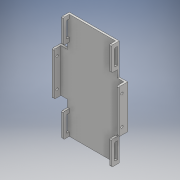
# Autodesk Inventor part: RCT-H112_stick_battery_plate
Saved by Autodesk Inventor 2018.1 (Build 221171000, 171)
## iProperties
Created: 2019-09-19
Part Number: RCT-H112_stick_battery_plate
Material: Generic
Document SubType Name: Modeling
Designer: maste
Density: 1 g/cm^3
Appearance: Default
Author: maste
Autodesk Inventor part; units mm, degrees
ref_plane "YZ Plane" through (0, 0, 0) normal (1, 0, 0) x (0, 1, 0)
ref_plane "XZ Plane" through (0, 0, 0) normal (0, 1, 0) x (-1, 0, 0)
ref_plane "XY Plane" through (0, 0, 0) normal (0, 0, 1) x (1, 0, 0)
sketch "Sketch1" plane through (0, 0, 0) normal (0, 1, 0) x (-1, 0, 0)
  line L0 (34.75, 22.5) -> (34.75, -22.5)
  line L1 (-34.75, 22.5) -> (-34.75, -22.5)
  line L2 (34.75, -22.5) -> (26, -22.5)
  line L3 (-34.75, -22.5) -> (-26, -22.5)
  line L4 (34.75, 22.5) -> (26, 22.5)
  line L5 (-34.75, 22.5) -> (-26, 22.5)
  line L6 (-26, -22.5) -> (-26, -55)
  line L7 (26, -22.5) -> (26, -55)
  line L8 (26, 22.5) -> (26, 55)
  line L9 (-26, 22.5) -> (-26, 55)
  line L10 (26, 55) -> (-26, 55)
  line L11 (26, -55) -> (-26, -55)
  point P0 (0, 0)
  dimension "d0" = 45
  dimension "d1" = 34.75
  dimension "d2" = 22.5
  dimension "d3" = 45
  dimension "d4" = 34.75
  dimension "d5" = 22.5
  dimension "d6" = 8.75
  dimension "d7" = 8.75
  dimension "d8" = 8.75
  dimension "d9" = 8.75
  dimension "d10" = 32.5
  dimension "d11" = 32.5
  dimension "d12" = 32.5
  dimension "d13" = 32.5
  constraints: 24 end point, 6 vertical, 4 horizontal
  measures "d0" distance of L0.start L0.end
  measures "d1" distance from line of point (0, 0) L0
  measures "d2" vertical distance of point (0, 0) L0.start
  measures "d3" distance of L1.start L1.end
  measures "d4" distance from line of point (0, 0) L1
  measures "d5" vertical distance of point (0, 0) L1.start
  measures "d6" distance of L0.end L2.end
  measures "d7" distance of L1.end L3.end
  measures "d8" distance of L0.start L4.end
  measures "d9" distance of L1.start L5.end
  measures "d10" distance of L3.end L6.end
  measures "d11" distance of L2.end L7.end
  measures "d12" distance of L4.end L8.end
  measures "d13" distance of L5.end L9.end
extrude "Extrusion1" add sketch "Sketch1" along normal blind 2
sketch "Sketch2" plane through (34.75, 0, 22.5) normal (1, 0, 0) x (0, 0, -1)
  line L0 (45, 2) -> (77.5, 2) projected
  line L1 (45, 2) -> (0, 2) projected
  line L2 (45, 2) -> (0, 2)
  line L3 (0, 2) -> (0, -6)
  line L4 (1, -7) -> (44, -7)
  line L5 (45, -6) -> (45, 2)
  line L6 (7.5, -4) -> (37.5, -4) construction
  circle A0 centre (7.5, -4) radius 1.25
  circle A1 centre (37.5, -4) radius 1.25
  arc A2 (0, -6) -> (1, -7) centre (1, -6) ccw
  arc A3 (44, -7) -> (45, -6) centre (44, -6) ccw
  point P0 (22.5, 0)
  point P1 (0, -7)
  point P2 (45, -7)
  dimension "d16" = 9
  dimension "d17" = 45
  dimension "d18" = 30
  dimension "d19" = 3
  dimension "d20" = 7.5
  dimension "d21" = 2.5
  dimension "d22" = 2.5
  dimension "d23" = 1
  dimension "d24" = 1
  constraints: 10 end point, 4 centre point, 4 point on circle, 4 point on line, 4 tangent, 2 coincident, 2 perpendicular, 1 collinear, 1 horizontal
  measures "d16" distance of L1.end point (0, -7)
  measures "d17" distance of point (0, -7) point (45, -7)
  measures "d18" distance of L6.start L6.end
  measures "d19" distance between parallel lines of L6 L4
  measures "d20" distance from line of L3 L6.start
  measures "d21" diameter of A0
  measures "d22" diameter of A1
  measures "d23" radius of A2
  measures "d24" radius of A3
extrude "Extrusion2" add sketch "Sketch2" against normal blind 2
sketch "Sketch3" plane through (-34.75, 0, -22.5) normal (-1, 0, 0) x (0, 0, 1)
  line L0 (-32.5, 2) -> (0, 2) projected
  line L1 (0, 2) -> (45, 2)
  line L2 (45, 2) -> (45, -6)
  line L3 (44, -7) -> (1, -7)
  line L4 (0, -6) -> (0, 2)
  circle A0 centre (37.5, -4) radius 1.25 projected
  circle A1 centre (37.5, -4) radius 1.25
  circle A2 centre (7.5, -4) radius 1.25 projected
  circle A3 centre (7.5, -4) radius 1.25
  arc A4 (0, -6) -> (1, -7) centre (1, -6) ccw
  arc A5 (44, -7) -> (45, -6) centre (44, -6) ccw
  point P0 (22.5, 0)
  point P1 (45, -7)
  point P2 (0, -7)
  dimension "d27" = 45
  dimension "d28" = 9
  dimension "d29" = 1
  constraints: 8 end point, 4 centre point, 4 point on circle, 4 point on line, 4 tangent, 2 coincident, 2 parallel, 1 equal radius, 1 horizontal, 1 perpendicular
  measures "d27" distance of point (45, -7) point (0, -7)
  measures "d28" distance of L1.end point (45, -7)
  measures "d29" radius of A4
extrude "Extrusion3" add sketch "Sketch3" against normal blind 2
sketch "Sketch4" plane through (26, 0, -22.5) normal (1, 0, 0) x (0, 0, -1)
  line L0 (32.5, 2) -> (0, 2) projected
  line L1 (7.5, 2) -> (7.5, -5)
  line L2 (8.5, -6) -> (31.5, -6)
  line L3 (32.5, -5) -> (32.5, 2)
  line L4 (12.5, -3) -> (27.5, -3)
  line L5 (11.5, -2) -> (11.5, 2)
  line L6 (28.5, -2) -> (28.5, 2)
  line L7 (32.5, 2) -> (28.5, 2)
  line L8 (11.5, 2) -> (7.5, 2)
  arc A0 (7.5, -5) -> (8.5, -6) centre (8.5, -5) ccw
  arc A1 (11.5, -2) -> (12.5, -3) centre (12.5, -2) ccw
  arc A2 (27.5, -3) -> (28.5, -2) centre (27.5, -2) ccw
  arc A3 (31.5, -6) -> (32.5, -5) centre (31.5, -5) ccw
  point P0 (-22.5, 0)
  point P1 (7.5, -6)
  point P2 (32.5, -6)
  point P3 (11.5, -3)
  point P4 (28.5, -3)
  dimension "d32" = 25
  dimension "d33" = 8
  dimension "d34" = 17
  dimension "d35" = 4
  dimension "d36" = 3
  dimension "d37" = 8
  dimension "d38" = 1
  constraints: 16 end point, 8 point on circle, 8 point on line, 8 tangent, 4 centre point, 4 perpendicular, 3 equal radius, 3 horizontal, 3 parallel
  measures "d32" distance of point (7.5, -6) point (32.5, -6)
  measures "d33" distance of point (32.5, -6) L0.start
  measures "d34" distance of point (11.5, -3) point (28.5, -3)
  measures "d35" distance from line of L1 point (11.5, -3)
  measures "d36" distance between parallel lines of L2 L4
  measures "d37" distance of L1.start point (7.5, -6)
  measures "d38" radius of A0
extrude "Extrusion4" add sketch "Sketch4" against normal blind 2 contours L3 A3 L2 A0 L1 L0 L5 A1 L4 A2 L6
sketch "Sketch5" plane through (26, 0, 55) normal (1, 0, 0) x (0, 0, -1)
  line L0 (0, 2) -> (32.5, 2) projected
  line L1 (25, 2) -> (25, -5)
  line L2 (24, -6) -> (1, -6)
  line L3 (0, -5) -> (0, 2)
  line L4 (5, -3) -> (20, -3)
  line L5 (4, -2) -> (4, 2)
  line L6 (21, -2) -> (21, 2)
  line L7 (0, 2) -> (4, 2)
  line L8 (21, 2) -> (25, 2)
  arc A0 (0, -5) -> (1, -6) centre (1, -5) ccw
  arc A1 (24, -6) -> (25, -5) centre (24, -5) ccw
  arc A2 (4, -2) -> (5, -3) centre (5, -2) ccw
  arc A3 (20, -3) -> (21, -2) centre (20, -2) ccw
  point P0 (55, 0)
  point P1 (25, -6)
  point P2 (0, -6)
  point P3 (4, -3)
  point P4 (21, -3)
  dimension "d41" = 25
  dimension "d42" = 8
  dimension "d43" = 17
  dimension "d44" = 5
  dimension "d45" = 4
  dimension "d46" = 8
  dimension "d47" = 1
  dimension "d65" = 1
  constraints: 16 end point, 8 point on circle, 8 point on line, 8 tangent, 4 centre point, 4 perpendicular, 3 horizontal, 3 parallel, 2 equal radius, 1 vertical
  measures "d41" distance of point (25, -6) point (0, -6)
  measures "d42" distance of point (0, -6) L0.start
  measures "d43" distance of point (4, -3) point (21, -3)
  measures "d44" distance between parallel lines of L0 L4
  measures "d45" distance from line of L3 point (4, -3)
  measures "d46" distance of L1.start point (25, -6)
  measures "d47" radius of A0
  measures "d65" radius of A2
extrude "Extrusion5" add sketch "Sketch5" against normal blind 2 contours L0 L5 A2 L4 A3 L6 L1 A1 L2 A0 L3
sketch "Sketch6" plane through (-26, 0, 22.5) normal (-1, 0, 0) x (0, 0, 1)
  line L0 (32.5, 0) -> (32.5, 2) projected
  line L1 (32.5, 2) -> (7.5, 2) construction
  line L2 (7.5, 2) -> (7.5, -5)
  line L3 (8.5, -6) -> (31.5, -6)
  line L4 (32.5, -5) -> (32.5, 2)
  line L5 (27.5, -3) -> (12.5, -3)
  line L6 (28.5, -2) -> (28.5, 2)
  line L7 (0, 2) -> (32.5, 2) projected
  line L8 (11.5, -2) -> (11.5, 2)
  line L9 (32.5, 2) -> (28.5, 2)
  line L10 (11.5, 2) -> (7.5, 2)
  arc A0 (31.5, -6) -> (32.5, -5) centre (31.5, -5) ccw
  arc A1 (7.5, -5) -> (8.5, -6) centre (8.5, -5) ccw
  arc A2 (11.5, -2) -> (12.5, -3) centre (12.5, -2) ccw
  arc A3 (27.5, -3) -> (28.5, -2) centre (27.5, -2) ccw
  line L11 (-77.5, 2) -> (-45, 2) construction
  line L12 (-77.5, 2) -> (-52.5, 2) construction
  line L13 (-52.5, 2) -> (-52.5, -5)
  line L14 (-53.5, -6) -> (-76.5, -6)
  line L15 (-77.5, -5) -> (-77.5, 2)
  line L16 (-57.5, -3) -> (-72.5, -3)
  line L17 (-56.5, -2) -> (-56.5, 2)
  line L18 (-73.5, -2) -> (-73.5, 2)
  line L19 (-52.5, 2) -> (-56.5, 2)
  line L20 (-73.5, 2) -> (-77.5, 2)
  arc A4 (-53.5, -6) -> (-52.5, -5) centre (-53.5, -5) ccw
  arc A5 (-57.5, -3) -> (-56.5, -2) centre (-57.5, -2) ccw
  arc A6 (-73.5, -2) -> (-72.5, -3) centre (-72.5, -2) ccw
  arc A7 (-77.5, -5) -> (-76.5, -6) centre (-76.5, -5) ccw
  point P0 (-22.5, 0)
  point P1 (7.5, -6)
  point P2 (32.5, -6)
  point P3 (28.5, -3)
  point P4 (11.5, -3)
  point P5 (-52.5, -6)
  point P6 (-77.5, -6)
  point P7 (-56.5, -3)
  point P8 (-73.5, -3)
  dimension "d50" = 25
  dimension "d51" = 8
  dimension "d52" = 17
  dimension "d53" = 4
  dimension "d54" = 3
  dimension "d55" = 1
  dimension "d56" = 1
  dimension "d57" = 1
  dimension "d58" = 1
  dimension "d59" = 25
  dimension "d60" = 8
  dimension "d61" = 17
  dimension "d62" = 4
  dimension "d63" = 3
  dimension "d64" = 1
  constraints: 36 end point, 20 point on line, 16 point on circle, 16 tangent, 8 centre point, 5 parallel, 4 collinear, 4 horizontal, 4 perpendicular, 3 equal radius, 1 vertical
  measures "d50" distance of point (7.5, -6) point (32.5, -6)
  measures "d51" distance of point (32.5, -6) L0.end
  measures "d52" distance of point (28.5, -3) point (11.5, -3)
  measures "d53" distance from line of L4 point (28.5, -3)
  measures "d54" distance between parallel lines of L3 L5
  measures "d55" radius of A0
  measures "d56" radius of A1
  measures "d57" radius of A2
  measures "d58" radius of A3
  measures "d59" distance of point (-52.5, -6) point (-77.5, -6)
  measures "d60" distance of point (-77.5, -6) L11.start
  measures "d61" distance of point (-56.5, -3) point (-73.5, -3)
  measures "d62" distance from line of L13 point (-56.5, -3)
  measures "d63" distance between parallel lines of L14 L16
  measures "d64" radius of A4
extrude "Extrusion6" add sketch "Sketch6" against normal blind 2 contours L4 A0 L3 A1 L2 L7 L8 A2 L5 A3 L6 L0 | L13 A4 L14 A7 L15 L20 L18 A6 L16 A5 L17 L19
body "Solid1"
